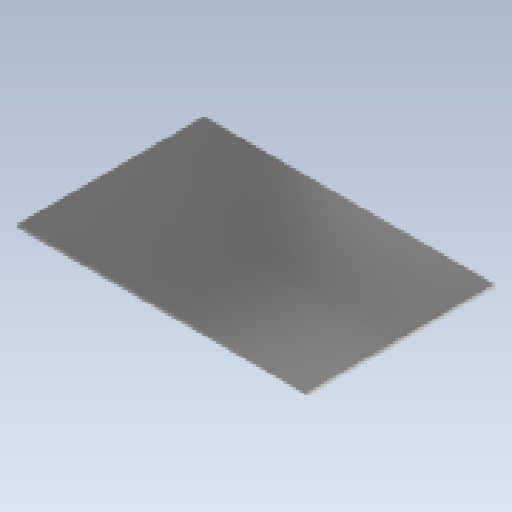
# Autodesk Inventor part: Платформа
Saved by Autodesk Inventor 2025.2 (Build 292293000, 293)
## iProperties
Created: 2025-01-21
Part Number: Платформа
Material: Нержавеющая сталь
Document SubType Name: Modeling
Designer: neket
Density: 8 g/cm^3
Appearance: С умеренной полировкой
Author: neket
Autodesk Inventor part; units mm, degrees
ref_plane "YZ Plane" through (0, 0, 0) normal (1, 0, 0) x (0, 1, 0)
ref_plane "XZ Plane" through (0, 0, 0) normal (0, 1, 0) x (-1, 0, 0)
ref_plane "XY Plane" through (0, 0, 0) normal (0, 0, 1) x (1, 0, 0)
sketch "Эскиз1" plane through (0, 0, 0) normal (0, 0, 1) x (1, 0, 0)
  line L0 (4, 0) -> (-276, 0)
  line L1 (-276, 0) -> (-276, 180)
  line L2 (-276, 180) -> (4, 180)
  line L3 (4, 180) -> (4, 0)
  point P0 (0, 0)
  dimension "d0" = 280
  dimension "d1" = 180
  constraints: 8 end point, 2 parallel, 1 horizontal, 1 perpendicular
  measures "d0" distance of L1.end L2.end
  measures "d1" distance of L0.end L1.end
extrude "Выдавливание1" add sketch "Эскиз1" along normal blind 3
